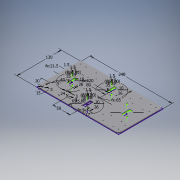
# Autodesk Inventor part: Base
Saved by Autodesk Inventor 2018 (Build 220112000, 112)
## iProperties
Created: 2021-04-30
Part Number: Base
Material: Generic
Document SubType Name: Modeling
Designer: dangl
Density: 1 g/cm^3
Appearance: Default
Author: dangl
Autodesk Inventor part; units mm, degrees
ref_plane "YZ Plane" through (0, 0, 0) normal (1, 0, 0) x (0, 1, 0)
ref_plane "XZ Plane" through (0, 0, 0) normal (0, 1, 0) x (-1, 0, 0)
ref_plane "XY Plane" through (0, 0, 0) normal (0, 0, 1) x (1, 0, 0)
sketch "Sketch1" plane through (0, 0, 0) normal (0, 1, 0) x (-1, 0, 0)
  line L0 (120, -65) -> (-120, -65)
  line L1 (-120, -65) -> (-120, 65)
  line L2 (-120, 65) -> (120, 65)
  line L3 (120, 65) -> (120, -65)
  circle A0 centre (65, 31) radius 1.5
  circle A1 centre (95, 31) radius 1.5
  circle A2 centre (65, 55) radius 1.5
  circle A3 centre (95, 55) radius 1.5
  line L4 (0, -65) -> (0, 65)
  line L5 (120, 0) -> (-120, 0)
  circle A4 centre (110, 55) radius 1.5
  circle A5 centre (110, 35) radius 1.5
  circle A6 centre (50, 40) radius 1.5
  circle A7 centre (65, -31) radius 1.5
  circle A8 centre (95, -31) radius 1.5
  circle A9 centre (65, -55) radius 1.5
  circle A10 centre (95, -55) radius 1.5
  circle A11 centre (110, -55) radius 1.5
  circle A12 centre (110, -35) radius 1.5
  circle A13 centre (50, -40) radius 1.5
  circle A14 centre (-65, 31) radius 1.5
  circle A15 centre (-95, 31) radius 1.5
  circle A16 centre (-65, 55) radius 1.5
  circle A17 centre (-95, 55) radius 1.5
  circle A18 centre (-110, 55) radius 1.5
  circle A19 centre (-110, 35) radius 1.5
  circle A20 centre (-50, 40) radius 1.5
  circle A21 centre (-95, -55) radius 1.5
  circle A22 centre (-65, -55) radius 1.5
  circle A23 centre (-50, -40) radius 1.5
  circle A24 centre (-110, -55) radius 1.5
  circle A25 centre (-110, -35) radius 1.5
  circle A26 centre (-95, -31) radius 1.5
  circle A27 centre (-65, -31) radius 1.5
  line L6 (110, -21.5) -> (110, -21.5)
  line L7 (108.5, -20) -> (108.5, 20)
  line L8 (110, 21.5) -> (110, 21.5)
  line L9 (111.5, 20) -> (111.5, -20)
  arc A28 (110, -21.5) -> (111.5, -20) centre (110, -20) ccw
  arc A29 (108.5, -20) -> (110, -21.5) centre (110, -20) ccw
  arc A30 (110, 21.5) -> (108.5, 20) centre (110, 20) ccw
  arc A31 (111.5, 20) -> (110, 21.5) centre (110, 20) ccw
  line L10 (-110, -21.5) -> (-110, -21.5)
  line L11 (-108.5, -20) -> (-108.5, 20)
  line L12 (-110, 21.5) -> (-110, 21.5)
  line L13 (-111.5, 20) -> (-111.5, -20)
  arc A32 (-111.5, -20) -> (-110, -21.5) centre (-110, -20) ccw
  arc A33 (-110, -21.5) -> (-108.5, -20) centre (-110, -20) ccw
  arc A34 (-108.5, 20) -> (-110, 21.5) centre (-110, 20) ccw
  arc A35 (-110, 21.5) -> (-111.5, 20) centre (-110, 20) ccw
  line L14 (3.5, 22) -> (-3.5, 22)
  line L15 (-5, 23.5) -> (-5, 46.5)
  line L16 (-3.5, 48) -> (3.5, 48)
  line L17 (5, 46.5) -> (5, 23.5)
  arc A36 (3.5, 22) -> (5, 23.5) centre (3.5, 23.5) ccw
  arc A37 (-5, 23.5) -> (-3.5, 22) centre (-3.5, 23.5) ccw
  arc A38 (-3.5, 48) -> (-5, 46.5) centre (-3.5, 46.5) ccw
  arc A39 (5, 46.5) -> (3.5, 48) centre (3.5, 46.5) ccw
  line L18 (5, 35) -> (-5, 35)
  line L19 (0, 35) -> (24.7487, 10.2513)
  line L20 (24.7487, 10.2513) -> (24.7487, 10.2513)
  line L21 (24.7487, 12.3726) -> (10.6066, 26.5147)
  line L22 (22.6274, 10.2513) -> (8.4853, 24.3934)
  line L23 (8.4853, 26.5147) -> (8.4853, 26.5147)
  arc A40 (22.6274, 10.2513) -> (24.7487, 10.2513) centre (23.6881, 11.3119) ccw
  arc A41 (24.7487, 10.2513) -> (24.7487, 12.3726) centre (23.6881, 11.3119) ccw
  arc A42 (8.4853, 26.5147) -> (8.4853, 24.3934) centre (9.5459, 25.4541) ccw
  arc A43 (10.6066, 26.5147) -> (8.4853, 26.5147) centre (9.5459, 25.4541) ccw
  line L24 (24.7487, 59.7487) -> (24.7487, 59.7487)
  arc A44 (24.7487, 59.7487) -> (22.6274, 59.7487) centre (23.6881, 58.6881) ccw
  arc A45 (24.7487, 57.6274) -> (24.7487, 59.7487) centre (23.6881, 58.6881) ccw
  line L25 (22.6274, 59.7487) -> (8.4853, 45.6066)
  line L26 (24.7487, 57.6274) -> (10.6066, 43.4853)
  arc A46 (8.4853, 45.6066) -> (8.4853, 43.4853) centre (9.5459, 44.5459) ccw
  line L27 (8.4853, 43.4853) -> (8.4853, 43.4853)
  arc A47 (8.4853, 43.4853) -> (10.6066, 43.4853) centre (9.5459, 44.5459) ccw
  line L28 (-24.7487, 59.7487) -> (-24.7487, 59.7487)
  arc A48 (-24.7487, 59.7487) -> (-24.7487, 57.6274) centre (-23.6881, 58.6881) ccw
  arc A49 (-22.6274, 59.7487) -> (-24.7487, 59.7487) centre (-23.6881, 58.6881) ccw
  line L29 (-24.7487, 57.6274) -> (-10.6066, 43.4853)
  line L30 (-22.6274, 59.7487) -> (-8.4853, 45.6066)
  arc A50 (-10.6066, 43.4853) -> (-8.4853, 43.4853) centre (-9.5459, 44.5459) ccw
  line L31 (-8.4853, 43.4853) -> (-8.4853, 43.4853)
  arc A51 (-8.4853, 43.4853) -> (-8.4853, 45.6066) centre (-9.5459, 44.5459) ccw
  line L32 (-24.7487, 10.2513) -> (-24.7487, 10.2513)
  arc A52 (-24.7487, 10.2513) -> (-22.6274, 10.2513) centre (-23.6881, 11.3119) ccw
  arc A53 (-24.7487, 12.3726) -> (-24.7487, 10.2513) centre (-23.6881, 11.3119) ccw
  line L33 (-22.6274, 10.2513) -> (-8.4853, 24.3934)
  line L34 (-24.7487, 12.3726) -> (-10.6066, 26.5147)
  arc A54 (-8.4853, 24.3934) -> (-8.4853, 26.5147) centre (-9.5459, 25.4541) ccw
  line L35 (-8.4853, 26.5147) -> (-8.4853, 26.5147)
  arc A55 (-8.4853, 26.5147) -> (-10.6066, 26.5147) centre (-9.5459, 25.4541) ccw
  line L36 (80, 0) -> (80, 10.2513)
  line L37 (83.5, -13) -> (76.5, -13)
  line L38 (75, -11.5) -> (75, 11.5)
  line L39 (76.5, 13) -> (83.5, 13)
  line L40 (85, 11.5) -> (85, -11.5)
  arc A56 (83.5, -13) -> (85, -11.5) centre (83.5, -11.5) ccw
  arc A57 (75, -11.5) -> (76.5, -13) centre (76.5, -11.5) ccw
  arc A58 (76.5, 13) -> (75, 11.5) centre (76.5, 11.5) ccw
  arc A59 (85, 11.5) -> (83.5, 13) centre (83.5, 11.5) ccw
  line L41 (85, 0) -> (75, 0)
  line L42 (80, 0) -> (104.7487, -24.7487)
  line L43 (104.7487, -24.7487) -> (104.7487, -24.7487)
  line L44 (104.7487, -22.6274) -> (90.6066, -8.4853)
  line L45 (102.6274, -24.7487) -> (88.4853, -10.6066)
  line L46 (88.4853, -8.4853) -> (88.4853, -8.4853)
  arc A60 (102.6274, -24.7487) -> (104.7487, -24.7487) centre (103.6881, -23.6881) ccw
  arc A61 (104.7487, -24.7487) -> (104.7487, -22.6274) centre (103.6881, -23.6881) ccw
  arc A62 (88.4853, -8.4853) -> (88.4853, -10.6066) centre (89.5459, -9.5459) ccw
  arc A63 (90.6066, -8.4853) -> (88.4853, -8.4853) centre (89.5459, -9.5459) ccw
  line L47 (104.7487, 24.7487) -> (104.7487, 24.7487)
  arc A64 (104.7487, 24.7487) -> (102.6274, 24.7487) centre (103.6881, 23.6881) ccw
  arc A65 (104.7487, 22.6274) -> (104.7487, 24.7487) centre (103.6881, 23.6881) ccw
  line L48 (102.6274, 24.7487) -> (88.4853, 10.6066)
  line L49 (104.7487, 22.6274) -> (90.6066, 8.4853)
  arc A66 (88.4853, 10.6066) -> (88.4853, 8.4853) centre (89.5459, 9.5459) ccw
  line L50 (88.4853, 8.4853) -> (88.4853, 8.4853)
  arc A67 (88.4853, 8.4853) -> (90.6066, 8.4853) centre (89.5459, 9.5459) ccw
  line L51 (55.2513, 24.7487) -> (55.2513, 24.7487)
  arc A68 (55.2513, 24.7487) -> (55.2513, 22.6274) centre (56.3119, 23.6881) ccw
  arc A69 (57.3726, 24.7487) -> (55.2513, 24.7487) centre (56.3119, 23.6881) ccw
  line L52 (55.2513, 22.6274) -> (69.3934, 8.4853)
  line L53 (57.3726, 24.7487) -> (71.5147, 10.6066)
  arc A70 (69.3934, 8.4853) -> (71.5147, 8.4853) centre (70.4541, 9.5459) ccw
  line L54 (71.5147, 8.4853) -> (71.5147, 8.4853)
  arc A71 (71.5147, 8.4853) -> (71.5147, 10.6066) centre (70.4541, 9.5459) ccw
  line L55 (55.2513, -24.7487) -> (55.2513, -24.7487)
  arc A72 (55.2513, -24.7487) -> (57.3726, -24.7487) centre (56.3119, -23.6881) ccw
  arc A73 (55.2513, -22.6274) -> (55.2513, -24.7487) centre (56.3119, -23.6881) ccw
  line L56 (57.3726, -24.7487) -> (71.5147, -10.6066)
  line L57 (55.2513, -22.6274) -> (69.3934, -8.4853)
  arc A74 (71.5147, -10.6066) -> (71.5147, -8.4853) centre (70.4541, -9.5459) ccw
  line L58 (71.5147, -8.4853) -> (71.5147, -8.4853)
  arc A75 (71.5147, -8.4853) -> (69.3934, -8.4853) centre (70.4541, -9.5459) ccw
  line L59 (-80, 0) -> (-80, 10.2513)
  arc A76 (-55.2513, -24.7487) -> (-55.2513, -22.6274) centre (-56.3119, -23.6881) ccw
  line L60 (-55.2513, -24.7487) -> (-55.2513, -24.7487)
  arc A77 (-57.3726, -24.7487) -> (-55.2513, -24.7487) centre (-56.3119, -23.6881) ccw
  line L61 (-55.2513, -22.6274) -> (-69.3934, -8.4853)
  line L62 (-71.5147, -8.4853) -> (-71.5147, -8.4853)
  arc A78 (-69.3934, -8.4853) -> (-71.5147, -8.4853) centre (-70.4541, -9.5459) ccw
  arc A79 (-71.5147, -8.4853) -> (-71.5147, -10.6066) centre (-70.4541, -9.5459) ccw
  line L63 (-57.3726, -24.7487) -> (-71.5147, -10.6066)
  arc A80 (-85, -11.5) -> (-83.5, -13) centre (-83.5, -11.5) ccw
  line L64 (-88.4853, -8.4853) -> (-88.4853, -8.4853)
  arc A81 (-88.4853, -10.6066) -> (-88.4853, -8.4853) centre (-89.5459, -9.5459) ccw
  arc A82 (-88.4853, -8.4853) -> (-90.6066, -8.4853) centre (-89.5459, -9.5459) ccw
  line L65 (-80, 0) -> (-104.7487, -24.7487)
  line L66 (-102.6274, -24.7487) -> (-88.4853, -10.6066)
  line L67 (-104.7487, -22.6274) -> (-90.6066, -8.4853)
  line L68 (-104.7487, -24.7487) -> (-104.7487, -24.7487)
  arc A83 (-104.7487, -24.7487) -> (-102.6274, -24.7487) centre (-103.6881, -23.6881) ccw
  arc A84 (-104.7487, -22.6274) -> (-104.7487, -24.7487) centre (-103.6881, -23.6881) ccw
  arc A85 (-83.5, 13) -> (-85, 11.5) centre (-83.5, 11.5) ccw
  arc A86 (-90.6066, 8.4853) -> (-88.4853, 8.4853) centre (-89.5459, 9.5459) ccw
  line L69 (-88.4853, 8.4853) -> (-88.4853, 8.4853)
  arc A87 (-88.4853, 8.4853) -> (-88.4853, 10.6066) centre (-89.5459, 9.5459) ccw
  line L70 (-104.7487, 22.6274) -> (-90.6066, 8.4853)
  arc A88 (-104.7487, 24.7487) -> (-104.7487, 22.6274) centre (-103.6881, 23.6881) ccw
  line L71 (-104.7487, 24.7487) -> (-104.7487, 24.7487)
  line L72 (-102.6274, 24.7487) -> (-88.4853, 10.6066)
  arc A89 (-102.6274, 24.7487) -> (-104.7487, 24.7487) centre (-103.6881, 23.6881) ccw
  arc A90 (-75, 11.5) -> (-76.5, 13) centre (-76.5, 11.5) ccw
  arc A91 (-71.5147, 10.6066) -> (-71.5147, 8.4853) centre (-70.4541, 9.5459) ccw
  line L73 (-71.5147, 8.4853) -> (-71.5147, 8.4853)
  arc A92 (-71.5147, 8.4853) -> (-69.3934, 8.4853) centre (-70.4541, 9.5459) ccw
  line L74 (-57.3726, 24.7487) -> (-71.5147, 10.6066)
  line L75 (-55.2513, 24.7487) -> (-55.2513, 24.7487)
  arc A93 (-55.2513, 24.7487) -> (-57.3726, 24.7487) centre (-56.3119, 23.6881) ccw
  arc A94 (-55.2513, 22.6274) -> (-55.2513, 24.7487) centre (-56.3119, 23.6881) ccw
  line L76 (-55.2513, 22.6274) -> (-69.3934, 8.4853)
  line L77 (-83.5, -13) -> (-76.5, -13)
  line L78 (-75, -11.5) -> (-75, 11.5)
  line L79 (-76.5, 13) -> (-83.5, 13)
  line L80 (-85, 11.5) -> (-85, -11.5)
  arc A95 (-76.5, -13) -> (-75, -11.5) centre (-76.5, -11.5) ccw
  line L81 (-85, 0) -> (-75, 0)
  line L82 (5, -35) -> (0, -35)
  line L83 (3.5, -48) -> (-3.5, -48)
  line L84 (-5, -46.5) -> (-5, -23.5)
  line L85 (-3.5, -22) -> (3.5, -22)
  line L86 (5, -23.5) -> (5, -46.5)
  arc A96 (3.5, -48) -> (5, -46.5) centre (3.5, -46.5) ccw
  arc A97 (-5, -46.5) -> (-3.5, -48) centre (-3.5, -46.5) ccw
  arc A98 (-3.5, -22) -> (-5, -23.5) centre (-3.5, -23.5) ccw
  arc A99 (5, -23.5) -> (3.5, -22) centre (3.5, -23.5) ccw
  line L87 (5, -35) -> (-5, -35)
  line L88 (0, -35) -> (24.7487, -59.7487)
  line L89 (24.7487, -59.7487) -> (24.7487, -59.7487)
  line L90 (24.7487, -57.6274) -> (10.6066, -43.4853)
  line L91 (22.6274, -59.7487) -> (8.4853, -45.6066)
  line L92 (8.4853, -43.4853) -> (8.4853, -43.4853)
  arc A100 (22.6274, -59.7487) -> (24.7487, -59.7487) centre (23.6881, -58.6881) ccw
  arc A101 (24.7487, -59.7487) -> (24.7487, -57.6274) centre (23.6881, -58.6881) ccw
  arc A102 (8.4853, -43.4853) -> (8.4853, -45.6066) centre (9.5459, -44.5459) ccw
  arc A103 (10.6066, -43.4853) -> (8.4853, -43.4853) centre (9.5459, -44.5459) ccw
  line L93 (24.7487, -10.2513) -> (24.7487, -10.2513)
  arc A104 (24.7487, -10.2513) -> (22.6274, -10.2513) centre (23.6881, -11.3119) ccw
  arc A105 (24.7487, -12.3726) -> (24.7487, -10.2513) centre (23.6881, -11.3119) ccw
  line L94 (22.6274, -10.2513) -> (8.4853, -24.3934)
  line L95 (24.7487, -12.3726) -> (10.6066, -26.5147)
  arc A106 (8.4853, -24.3934) -> (8.4853, -26.5147) centre (9.5459, -25.4541) ccw
  line L96 (8.4853, -26.5147) -> (8.4853, -26.5147)
  arc A107 (8.4853, -26.5147) -> (10.6066, -26.5147) centre (9.5459, -25.4541) ccw
  line L97 (-24.7487, -10.2513) -> (-24.7487, -10.2513)
  arc A108 (-24.7487, -10.2513) -> (-24.7487, -12.3726) centre (-23.6881, -11.3119) ccw
  arc A109 (-22.6274, -10.2513) -> (-24.7487, -10.2513) centre (-23.6881, -11.3119) ccw
  line L98 (-24.7487, -12.3726) -> (-10.6066, -26.5147)
  line L99 (-22.6274, -10.2513) -> (-8.4853, -24.3934)
  arc A110 (-10.6066, -26.5147) -> (-8.4853, -26.5147) centre (-9.5459, -25.4541) ccw
  line L100 (-8.4853, -26.5147) -> (-8.4853, -26.5147)
  arc A111 (-8.4853, -26.5147) -> (-8.4853, -24.3934) centre (-9.5459, -25.4541) ccw
  line L101 (-24.7487, -59.7487) -> (-24.7487, -59.7487)
  arc A112 (-24.7487, -59.7487) -> (-22.6274, -59.7487) centre (-23.6881, -58.6881) ccw
  arc A113 (-24.7487, -57.6274) -> (-24.7487, -59.7487) centre (-23.6881, -58.6881) ccw
  line L102 (-22.6274, -59.7487) -> (-8.4853, -45.6066)
  line L103 (-24.7487, -57.6274) -> (-10.6066, -43.4853)
  arc A114 (-8.4853, -45.6066) -> (-8.4853, -43.4853) centre (-9.5459, -44.5459) ccw
  line L104 (-8.4853, -43.4853) -> (-8.4853, -43.4853)
  arc A115 (-8.4853, -43.4853) -> (-10.6066, -43.4853) centre (-9.5459, -44.5459) ccw
  point P0 (0, 0)
  point P1 (5, 22)
  point P2 (-5, 48)
  point P3 (-5, 22)
  point P4 (23.6881, 9.1906)
  point P5 (25.8094, 11.3119)
  point P6 (7.4246, 25.4541)
  point P7 (23.6881, 60.8094)
  point P8 (24.7487, 59.7487)
  point P9 (25.8094, 58.6881)
  point P10 (9.5459, 42.4246)
  point P11 (-25.8094, 58.6881)
  point P12 (-24.7487, 59.7487)
  point P13 (-23.6881, 60.8094)
  point P14 (-7.4246, 44.5459)
  point P15 (-23.6881, 9.1906)
  point P16 (-24.7487, 10.2513)
  point P17 (-25.8094, 11.3119)
  point P18 (-9.5459, 27.5754)
  point P19 (85, -13)
  point P20 (75, 13)
  point P21 (75, -13)
  point P22 (103.6881, -25.8094)
  point P23 (105.8094, -23.6881)
  point P24 (87.4246, -9.5459)
  point P25 (103.6881, 25.8094)
  point P26 (104.7487, 24.7487)
  point P27 (105.8094, 23.6881)
  point P28 (89.5459, 7.4246)
  point P29 (54.1906, 23.6881)
  point P30 (56.3119, 25.8094)
  point P31 (72.5754, 9.5459)
  point P32 (56.3119, -25.8094)
  point P33 (55.2513, -24.7487)
  point P34 (54.1906, -23.6881)
  point P35 (70.4541, -7.4246)
  point P36 (-54.1906, -23.6881)
  point P37 (-55.2513, -24.7487)
  point P38 (-56.3119, -25.8094)
  point P39 (-70.4541, -7.4246)
  point P40 (-85, -13)
  point P41 (-87.4246, -9.5459)
  point P42 (-103.6881, -25.8094)
  point P43 (-105.8094, -23.6881)
  point P44 (-89.5459, 7.4246)
  point P45 (-105.8094, 23.6881)
  point P46 (-104.7487, 24.7487)
  point P47 (-103.6881, 25.8094)
  point P48 (-75, 13)
  point P49 (-72.5754, 9.5459)
  point P50 (-56.3119, 25.8094)
  point P51 (-54.1906, 23.6881)
  point P52 (-75, -13)
  point P53 (-5, -35)
  point P54 (5, -48)
  point P55 (-5, -22)
  point P56 (-5, -48)
  point P57 (23.6881, -60.8094)
  point P58 (25.8094, -58.6881)
  point P59 (7.4246, -44.5459)
  point P60 (23.6881, -9.1906)
  point P61 (24.7487, -10.2513)
  point P62 (25.8094, -11.3119)
  point P63 (9.5459, -27.5754)
  point P64 (-25.8094, -11.3119)
  point P65 (-24.7487, -10.2513)
  point P66 (-23.6881, -9.1906)
  point P67 (-7.4246, -25.4541)
  point P68 (-23.6881, -60.8094)
  point P69 (-24.7487, -59.7487)
  point P70 (-25.8094, -58.6881)
  point P71 (-9.5459, -42.4246)
  dimension "d4" = 240
  dimension "d5" = 130
  dimension "d6" = 65
  dimension "d7" = 120
  dimension "d8" = 3
  dimension "d9" = 65
  dimension "d10" = 31
  dimension "d13" = 30
  dimension "d16" = 24
  dimension "d19" = 3
  dimension "d20" = 15
  dimension "d21" = 3
  dimension "d22" = 20
  dimension "d23" = 3
  dimension "d24" = 50
  dimension "d26" = 25
  dimension "d27" = 43
  dimension "d28" = 21.5
  dimension "d29" = 1.5
  dimension "d30" = 10
  dimension "d31" = 26
  dimension "d32" = 17
  dimension "d33" = 5
  dimension "d34" = 1.5
  dimension "d35" = 45
  dimension "d36" = 35
  dimension "d38" = 3
  dimension "d39" = 1.5
  dimension "d40" = 23
  dimension "d41" = 1.5
  dimension "d44" = 360
  dimension "d46" = 80
  dimension "d53" = 10
  dimension "d54" = 26
  dimension "d55" = 1.5
  dimension "d56" = 35
  dimension "d57" = 3
  dimension "d58" = 1.5
  dimension "d59" = 23
  dimension "d60" = 1.5
  dimension "d61" = 360
  dimension "d72" = 10
  dimension "d73" = 26
  dimension "d74" = 1.5
  dimension "d75" = 35
  dimension "d76" = 3
  dimension "d77" = 1.5
  dimension "d78" = 23
  dimension "d79" = 1.5
  dimension "d80" = 360
  constraints: 210 end point, 176 point on circle, 122 point on line, 119 symmetric about line, 116 centre point, 58 tangent, 21 equal radius, 13 midpoint, 11 perpendicular, 10 parallel, 6 horizontal, 2 vertical, 342 other
  measures "d4" distance of L0.start L0.end
  measures "d5" distance of L2.end L0.start
  measures "d6" distance from line of point (0, 0) L0
  measures "d7" distance from line of L3 point (0, 0)
  measures "d8" diameter of A0
  measures "d9" horizontal distance of A0.centre point (0, 0)
  measures "d10" vertical distance of A0.centre point (0, 0)
  measures "d13" distance of A0.centre A1.centre
  measures "d16" distance of A0.centre A2.centre
  measures "d19" diameter of A4
  measures "d20" distance of A3.centre A4.centre
  measures "d21" diameter of A5
  measures "d22" distance of A4.centre A5.centre
  measures "d23" diameter of A6
  measures "d24" horizontal distance of point (0, 0) A6.centre
  measures "d26" distance from line of L2 A6.centre
  measures "d27" distance between parallel lines of L8 L6
  measures "d28" distance between parallel lines of L5 L6
  measures "d29" radius of A28
  measures "d30" distance of point (5, 22) point (-5, 22)
  measures "d31" distance of point (-5, 22) point (-5, 48)
  measures "d32" distance between parallel lines of L2 L16
  measures "d33" distance from line of point (0, 0) L15
  measures "d34" radius of A36
  measures "d35" angle of L2 L19
  measures "d36" distance of L19.start L19.end
  measures "d38" distance of point (23.688, 9.191) point (25.809, 11.312)
  measures "d39" distance between parallel lines of L19 L22
  measures "d40" distance of point (23.688, 9.191) point (7.425, 25.454)
  measures "d41" radius of A40
  measures "d46" distance between parallel lines of L4 L36
  measures "d53" distance of point (85, -13) point (75, -13)
  measures "d54" distance of point (75, -13) point (75, 13)
  measures "d55" radius of A56
  measures "d56" distance of L42.start L42.end
  measures "d57" distance of point (103.688, -25.809) point (105.809, -23.688)
  measures "d58" distance between parallel lines of L42 L45
  measures "d59" distance of point (103.688, -25.809) point (87.425, -9.546)
  measures "d60" radius of A60
  measures "d72" distance of point (5, -48) point (-5, -48)
  measures "d73" distance of point (-5, -48) point (-5, -22)
  measures "d74" radius of A96
  measures "d75" distance of L88.start L88.end
  measures "d76" distance of point (23.688, -60.809) point (25.809, -58.688)
  measures "d77" distance between parallel lines of L88 L91
  measures "d78" distance of point (23.688, -60.809) point (7.425, -44.546)
  measures "d79" radius of A100
extrude "Extrusion2" add sketch "Sketch1" along normal blind 3 contours L0 L4 L83 A96 L86 A99 L85 L5 L38 A57 L37 A56 L40 L7 A29 A28 L9 L3 | L0 L1 L5 L13 A32 A33 L11 L80 A80 L77 A95 L78 L4 L85 A98 L84 A97 L83 | L5 L9 A31 A30 L7 L40 A59 L39 A58 L38 L4 L14 A36 L17 A39 L16 L2 L3 | L9 A28 A29 L7 L5 | L5 L7 A30 A31 L9 | L1 L2 L4 L16 A38 L15 A37 L14 L5 L78 A90 L79 A85 L80 L11 A34 A35 L13 | L13 A35 A34 L11 L5 | L5 L11 A33 A32 L13
fillet "Fillet1" radius 10 4 edges at (-120, 1.5, -65) (-120, 1.5, 65) (120, 1.5, 65) (120, 1.5, -65)
equation "\"d6\" = 0.5 * d5"
equation "\"d7\" = 0.5 * d4"
equation "\"d28\" = 0.5 * d27"
equation "\"d33\" = 0.5 * d30"
equation "\"d39\" = 0.5 * d38"
equation "\"d58\" = 0.5 * d57"
equation "\"d77\" = 0.5 * d76"
body "Solid1"
